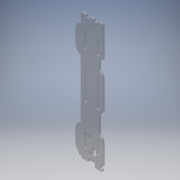
# Autodesk Inventor part: Left_wall
Saved by Autodesk Inventor 2016 (Build 200138000, 138)
## iProperties
Created: 2015-06-19
Part Number: Left_wall
Material: Generic
Document SubType Name: Modeling
Designer: Openlab
Density: 1 g/cm^3
Appearance: Polycarbonate - Clear
Author: Openlab
Autodesk Inventor part; units mm, degrees
ref_plane "YZ Plane" through (0, 0, 0) normal (1, 0, 0) x (0, 1, 0)
ref_plane "XZ Plane" through (0, 0, 0) normal (0, 1, 0) x (-1, 0, 0)
ref_plane "XY Plane" through (0, 0, 0) normal (0, 0, 1) x (1, 0, 0)
sketch "Sketch1" plane through (0, 0, 0) normal (0, 1, 0) x (-1, 0, 0)
  line L0 (26.5, -25) -> (23.5, -25)
  line L1 (26.5, -43) -> (23.5, -43)
  line L2 (26.5, -68.5) -> (23.5, -68.5)
  line L3 (26.5, -109.5) -> (23.5, -109.5)
  line L4 (8, -68.5) -> (5, -68.5)
  line L5 (8, -109.5) -> (5, -109.5)
  line L6 (8, -43) -> (5, -43)
  line L7 (8, -25) -> (5, -25)
  line L8 (23.5, -109.5) -> (23.5, -68.5)
  line L9 (23.5, -43) -> (23.5, -25)
  line L10 (8, -109.5) -> (8, -68.5)
  line L11 (8, -43) -> (8, -25)
  line L12 (8, -167) -> (8, -149)
  line L13 (26.5, -149) -> (23.5, -149)
  line L14 (8, -149) -> (5, -149)
  line L15 (23.5, -149) -> (23.5, -167)
  line L16 (23.5, -167) -> (26.5, -167)
  line L17 (5, -167) -> (8, -167)
  line L18 (20.5, -169) -> (18.7, -169)
  line L19 (18.7, -169) -> (18.7, -174)
  line L20 (18.7, -174) -> (20.5, -174)
  line L21 (20.5, -174) -> (20.5, -169)
  line L22 (15.75, -110.2512) -> (15.75, -143.2512) construction
  line L23 (26.5, -25) -> (26.5, -43)
  line L24 (26.5, -68.5) -> (26.5, -109.5)
  line L25 (26.5, -149) -> (26.5, -167)
  line L26 (5, -167) -> (5, -149)
  line L27 (5, -109.5) -> (5, -68.5)
  line L28 (5, -43) -> (5, -25)
  line L29 (12.25, -3) -> (8, -3)
  line L30 (19.25, -3) -> (19.25, 0)
  line L31 (19.25, 0) -> (12.25, 0)
  line L32 (12.25, 0) -> (12.25, -3)
  line L33 (19.25, -3) -> (23.5, -3)
  line L34 (3.5, -179) -> (3.5, -182)
  line L35 (11, -179) -> (20.5, -179)
  line L36 (20.5, -179) -> (20.5, -182)
  line L37 (20.5, -182) -> (30.3328, -182)
  line L38 (30.5, -179) -> (31.5, -179)
  line L39 (3.5, -182) -> (1.5, -182)
  line L40 (23.5, -3) -> (23.5, 0)
  line L41 (23.5, 0) -> (28.5, 0)
  line L42 (8, -3) -> (8, 0)
  line L43 (8, 0) -> (3, 0)
  line L44 (1.5, -185) -> (10.5394, -185)
  arc A0 (30.3328, -182) -> (30.5, -179) centre (3.5, -179) ccw
  arc A1 (5, -141.5838) -> (0, -149) centre (8, -149) ccw
  arc A2 (5, -61.0838) -> (0, -68.5) centre (8, -68.5) ccw
  line L45 (5, -50.4162) -> (5, -61.0838)
  line L46 (5, -116.9162) -> (5, -141.5838)
  line L47 (19.5, -129.25) -> (13.2, -129.25) construction
  arc A3 (0, -109.5) -> (5, -116.9162) centre (8, -109.5) ccw
  line L48 (0, -177.9348) -> (0, -149)
  arc A4 (0, -43) -> (5, -50.4162) centre (8, -43) ccw
  line L49 (0, -109.5) -> (0, -68.5)
  line L50 (0, -43) -> (0, -3)
  arc A5 (31.5, -54.4564) -> (39, -43) centre (26.5, -43) ccw
  line L51 (39, -25) -> (39, -43)
  arc A6 (39, -25) -> (31.5, -13.5436) centre (26.5, -25) ccw
  line L52 (31.5, -3) -> (31.5, -13.5436)
  arc A7 (39, -149) -> (31.5, -137.5436) centre (26.5, -149) ccw
  line L53 (39, -167) -> (39, -149)
  arc A8 (34, -177) -> (39, -167) centre (26.5, -167) ccw
  line L54 (31.5, -54.4564) -> (31.5, -137.5436)
  arc A9 (31.5, -3) -> (28.5, 0) centre (28.5, -3) ccw
  arc A10 (3, 0) -> (0, -3) centre (3, -3) ccw
  line L55 (20.5, -149) -> (18.7, -149)
  line L56 (18.7, -149) -> (18.7, -154)
  line L57 (18.7, -154) -> (20.5, -154)
  line L58 (20.5, -154) -> (20.5, -149)
  line L59 (15, -163) -> (10, -163)
  line L60 (10, -163) -> (10, -171)
  line L61 (10, -171) -> (15, -171)
  line L62 (15, -171) -> (15, -163)
  line L63 (12.5, -163.9683) -> (12.5, -168.686) construction
  line L64 (14.8699, -167) -> (11.7199, -167) construction
  arc A11 (10.5394, -185) -> (11, -182) centre (1, -182) ccw
  line L65 (11, -182) -> (11, -179)
  line L66 (13.5, -179) -> (13.5, -182) construction
  line L67 (13.5, -182) -> (3.5, -182) construction
  line L68 (30.5, -179) -> (30.5, -182) construction
  line L69 (30.5, -182) -> (30.3328, -182) construction
  line L70 (31.5, -179) -> (34, -179)
  line L71 (34, -179) -> (34, -177)
  line L72 (31.5, -179) -> (31.5, -174.1753) construction
  line L73 (26.5, -179) -> (26.5, -186) construction
  line L74 (26.5, -186) -> (23.5, -186) construction
  line L75 (23.5, -186) -> (23.5, -179) construction
  line L76 (30.5, -179) -> (20.5, -179) construction
  line L77 (3.5, -179) -> (0, -177.9348)
  line L78 (1, -182.5) -> (1, -184.5)
  arc A12 (1.5, -182) -> (1, -182.5) centre (1.5, -182.5) ccw
  arc A13 (1, -184.5) -> (1.5, -185) centre (1.5, -184.5) ccw
  point P0 (0, 0)
  point P1 (1, -185)
  point P2 (1, -182)
  dimension "d7" = 18
  dimension "d8" = 25.5
  dimension "d9" = 41
  dimension "d39" = 18
  dimension "d45" = 5
  dimension "d56" = 3
  dimension "d61" = 39.5
  dimension "d62" = 15.5
  dimension "d64" = 12
  dimension "d65" = 7
  dimension "d74" = 176
  dimension "d75" = 15.5
  dimension "d85" = 10
  dimension "d90" = 5
  dimension "d92" = 25
  dimension "d104" = 6
  dimension "d105" = 5
  dimension "d106" = 1.8
  dimension "d107" = 3
  dimension "d108" = 15
  dimension "d110" = 8
  dimension "d111" = 5
  dimension "d112" = 8
  dimension "d113" = 12
  dimension "d114" = 7
  dimension "d115" = 10
  dimension "d116" = 3
  dimension "d121" = 2.5
  dimension "d122" = 25
  dimension "d123" = 7
  dimension "d124" = 10
  dimension "d125" = 2.5
  dimension "d126" = 2.5
  dimension "d127" = 0.5
  constraints: 159 end point, 28 point on circle, 26 collinear, 23 tangent, 22 point on line, 14 centre point, 14 perpendicular, 14 vertical, 9 equal length, 8 horizontal, 7 coincident, 7 parallel, 5 equal radius, 8 other
  measures "d7" distance between parallel lines of L1 L0
  measures "d8" distance between parallel lines of L2 L1
  measures "d9" distance between parallel lines of L3 L2
  measures "d39" distance of L13.end L15.end
  measures "d45" distance of L20.end L18.start
  measures "d56" distance of L0.start L0.end
  measures "d61" distance between parallel lines of L3 L13
  measures "d62" distance between parallel lines of L10 L8
  measures "d64" distance between parallel lines of L16 L38
  measures "d65" distance of L30.end L31.end
  measures "d74" distance between parallel lines of L38 L33
  measures "d75" distance between parallel lines of L42 L40
  measures "d85" distance from line of L38.start L36
  measures "d90" distance between parallel lines of L48 L26
  measures "d92" diameter of A5
  measures "d104" diameter of A9
  measures "d105" distance between parallel lines of L20 L35
  measures "d106" distance of L55.start L55.end
  measures "d107" distance between parallel lines of L58 L15
  measures "d108" distance between parallel lines of L18 L57
  measures "d110" distance of L59.end L60.end
  measures "d111" distance of L59.start L59.end
  measures "d112" distance between parallel lines of L63 L21
  measures "d113" distance between parallel lines of L35 L64
  measures "d114" distance between parallel lines of L66 L36
  measures "d115" distance between parallel lines of L34 L66
  measures "d116" distance between parallel lines of L39 L44
  measures "d121" distance of L38.end L70.end
  measures "d122" distance between parallel lines of L0 L41
  measures "d123" distance of L73.start L73.end
  measures "d124" distance between parallel lines of L78 L65
  measures "d125" distance between parallel lines of L65 L66
  measures "d126" distance of L34.end point (1, -182)
  measures "d127" radius of A12
extrude "Extrusion3" add sketch "Sketch1" along normal blind 3
body "Solid3"
